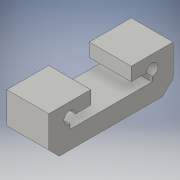
# Autodesk Inventor part: led_clip_v2
Saved by Autodesk Inventor 2016 (Build 200138000, 138)
## iProperties
Created: 2016-02-27
Part Number: led_clip_v2
Material: Generic
Document SubType Name: Modeling
Designer: Matt Ruffner
Density: 1 g/cm^3
Appearance: Default
Author: Matt Ruffner
Autodesk Inventor part; units mm, degrees
ref_plane "YZ Plane" through (0, 0, 0) normal (1, 0, 0) x (0, 1, 0)
ref_plane "XZ Plane" through (0, 0, 0) normal (0, 1, 0) x (-1, 0, 0)
ref_plane "XY Plane" through (0, 0, 0) normal (0, 0, 1) x (1, 0, 0)
sketch "Sketch1" plane through (0, 0, 0) normal (1, 0, 0) x (0, 1, 0)
  arc A0 (0, 16.1546) -> (-0.889, 17.0436) centre (0, 17.0436) ccw
  arc A1 (-0.889, 4.5468) -> (0, 5.4358) centre (0, 4.5468) ccw
  line L0 (0, 13.8686) -> (2.0409, 13.8686)
  line L1 (0, 7.7218) -> (2.0409, 7.7218)
  line L2 (2.0409, 7.7218) -> (2.0409, 1.3718)
  line L3 (2.0409, 1.3718) -> (-2.7216, 1.3718)
  line L4 (2.0409, 13.8686) -> (2.0409, 20.2186)
  line L5 (2.0409, 20.2186) -> (-2.7216, 20.2186)
  line L6 (-4.3091, 18.6311) -> (-4.3091, 2.9593)
  line L7 (-2.7216, 20.2186) -> (-4.3091, 18.6311)
  line L8 (-2.7216, 1.3718) -> (-4.3091, 2.9593)
  line L9 (0, 3.6578) -> (-1.5964, 3.6578)
  line L10 (-1.5964, 4.5468) -> (-1.5964, 17.0436)
  line L11 (-1.5964, 17.9326) -> (0, 17.9326)
  line L12 (0, 16.1546) -> (0, 13.8686)
  line L13 (0, 7.7218) -> (0, 5.4358)
  line L14 (-0.889, 4.5468) -> (-1.5964, 4.5468)
  line L15 (-0.889, 17.0436) -> (-1.5964, 17.0436)
  point P0 (0, 0)
  point P1 (-4.3091, 1.3718)
  point P2 (-4.3091, 20.2186)
  dimension "d0" = 14.2748
  dimension "d1" = 1.778
  dimension "d2" = 0.889
  dimension "d3" = 1.778
  dimension "d4" = 0.889
  dimension "d5" = 3.175
  dimension "d6" = 3.175
  dimension "d7" = 6.35
  dimension "d8" = 6.35
  dimension "d9" = 6.35
  dimension "d10" = 1.5875
  dimension "d11" = 1.5875
  dimension "d12" = 1.5875
  dimension "d13" = 1.5875
  constraints: 32 end point, 6 perpendicular, 6 point on line, 4 point on circle, 4 vertical, 3 horizontal, 2 centre point, 1 tangent
  measures "d0" distance of L11.end L9.start
  measures "d1" diameter of A0
  measures "d2" distance of L11.end A0.centre
  measures "d3" diameter of A1
  measures "d4" distance of L9.start A1.centre
  measures "d5" distance of A0.centre L0.start
  measures "d6" distance from line of A1.centre L1
  measures "d7" distance of L1.end L2.end
  measures "d8" distance of L2.end point (-4.309, 1.372)
  measures "d9" distance of L0.end L4.end
  measures "d10" distance of L5.end point (-4.309, 20.219)
  measures "d11" distance of L6.start point (-4.309, 20.219)
  measures "d12" distance of L3.end point (-4.309, 1.372)
  measures "d13" distance of L6.end point (-4.309, 1.372)
extrude "Extrusion1" add sketch "Sketch1" along normal blind 6.35
equation "\"d11\" = d10"
equation "\"d12\" = d10"
equation "\"d13\" = d12"
body "Solid1"
